remotethumbstick (Autodesk Fusion 360 design; units mm, degrees)
Autodesk Fusion 360 part; units mm, degrees
note: some values were not read from the file. Chosen so that the rebuilt part matches the saved one: which face or edge a step refers to.
sketch "Sketch1" plane through (0, 0, 0) normal (0, 1, 0) x (1, 0, 0)
  line L0 (0, 0) -> (-13.2, 0)
  line L1 (-13.2, 0) -> (-13.2, -13.2)
  line L2 (-13.2, -13.2) -> (0, -13.2)
  line L3 (0, -13.2) -> (0, 0)
  dimension "d1" = 13.2
  dimension "d2" = 13.2
  constraint horizontal L0
  constraint vertical L1
  constraint horizontal L2
  constraint vertical L3
  constraint coincident L0.start L3.end
  measures "d1" distance of L1.end L2.end
  measures "d2" distance of L0.end L1.end
extrude "Extrude1" add sketch "Sketch1" along normal blind 12 makes body 1
sketch "Sketch3" plane through (0, 0, 0) normal (0, 0, -1) x (1, 0, 0)
  line L0 (0, 0) -> (-13.2, 0)
  line L1 (-13.2, 0) -> (-13.2, -12)
  line L2 (-13.2, -12) -> (0, -12)
  line L3 (0, -12) -> (0, 0)
  line L4 (-11.4, 0) -> (-1.8, 0)
  line L5 (-1.8, 0) -> (-1.8, -12)
  line L6 (-1.8, -12) -> (-11.4, -12)
  line L7 (-11.4, -12) -> (-11.4, 0)
  dimension "d10" = 9.6
  dimension "d11" = 1.8
  constraint horizontal L4
  constraint vertical L5
  constraint horizontal L6
  constraint vertical L7
  constraint coincident L2 L5.end
  constraint coincident L0 L4.start
  measures "d10" distance of L4.start L4.end
  measures "d11" distance of L3 L5
extrude "Extrude3" add sketch "Sketch3" along normal blind 3 contours L0 L2 L4 L5 L6 L7 bodies 1
sketch "Sketch4" plane through (-13.2, 0, 0) normal (-1, 0, 0) x (0, -1, 0)
  line L0 (0, 0) -> (0, 13.2)
  line L1 (0, 13.2) -> (-12, 13.2)
  line L2 (-12, 13.2) -> (-12, 0)
  line L3 (-12, 0) -> (0, 0)
  line L4 (-12, 11.4) -> (0, 11.4)
  line L5 (0, 11.4) -> (0, 1.8)
  line L6 (0, 1.8) -> (-12, 1.8)
  line L7 (-12, 1.8) -> (-12, 11.4)
  dimension "d14" = 1.8
  dimension "d15" = 1.8
  constraint horizontal L4
  constraint vertical L5
  constraint horizontal L6
  constraint vertical L7
  constraint coincident L0 L5.end
  constraint coincident L2 L4.start
  measures "d14" distance of L1 L4
  measures "d15" distance of L3 L6
extrude "Extrude4" add sketch "Sketch4" along normal blind 3 contours L0 L2 L4 L5 L6 L7 bodies 1
sketch "Sketch6" plane through (0, 0, 13.2) normal (0, 0, 1) x (-1, 0, 0)
  line L0 (13.2, 0) -> (0, 0)
  line L1 (0, 0) -> (0, -12)
  line L2 (0, -12) -> (13.2, -12)
  line L3 (13.2, -12) -> (13.2, 0)
  line L4 (10.9, 0) -> (2.3, 0)
  line L5 (2.3, 0) -> (2.3, -5)
  line L6 (2.3, -5) -> (10.9, -5)
  line L7 (10.9, -5) -> (10.9, 0)
  dimension "d22" = 5
  dimension "d23" = 8.6
  dimension "d24" = 2.3
  constraint horizontal L4
  constraint vertical L5
  constraint horizontal L6
  constraint vertical L7
  constraint coincident L0 L4.start
  measures "d22" distance of L4.start L6.end
  measures "d23" distance of L4.start L4.end
  measures "d24" distance of L3 L7
extrude "Extrude6" [suppressed]
sketch "Sketch7" plane through (-10.9, 0, 0) normal (-1, 0, 0) x (0, -1, 0)
  line L0 (-5, 13.2) -> (0, 13.2)
  line L1 (0, 13.2) -> (0, 18.2)
  line L2 (0, 18.2) -> (-5, 18.2)
  line L3 (-5, 18.2) -> (-5, 13.2)
  line L4 (-5, 16.8629) -> (-8.201, 13.1133)
  line L5 (-5, 16.8629) -> (-5, 13.2)
  line L6 (-8.201, 13.1133) -> (-5, 13.2)
  point P0 (-12, 13.2)
  dimension "d27" = 3.8
  constraint coincident L3 L4.start
  constraint coincident L0.start L3.end
  measures "d27" distance of L4.end P0
extrude "Extrude7" [suppressed]
sketch "Sketch8" plane through (0, 0, 0) normal (1, 0, 0) x (0, 1, 0)
  line L0 (0, 13.2) -> (0, 0)
  line L1 (0, 0) -> (12, 0)
  line L2 (12, 0) -> (12, 13.2)
  line L3 (12, 13.2) -> (0, 13.2)
  line L4 (0, 10.9) -> (5, 10.9)
  line L5 (5, 10.9) -> (5, 2.3)
  line L6 (5, 2.3) -> (0, 2.3)
  line L7 (0, 2.3) -> (0, 10.9)
  dimension "d30" = 8.6
  dimension "d31" = 2.3
  dimension "d34" = 5
  constraint horizontal L4
  constraint vertical L5
  constraint horizontal L6
  constraint vertical L7
  constraint coincident L0 L4.start
  measures "d30" distance of L4.start L6.end
  measures "d31" distance of L3 L4
  measures "d34" distance of L5.end L6.end
extrude "Extrude8" add sketch "Sketch8" along normal blind 5 contours L0 L4 L5 L6 L7 bodies 1
sketch "Sketch9" plane through (0, 0, 10.9) normal (0, 0, 1) x (-1, 0, 0)
  line L0 (0, -5) -> (0, 0)
  line L1 (0, 0) -> (-5, 0)
  line L2 (-5, 0) -> (-5, -5)
  line L3 (-5, -5) -> (0, -5)
  line L4 (-3.7501, -5) -> (0, -8.4788)
  line L5 (0, -8.4788) -> (0, -5)
  line L6 (-3.7501, -5) -> (0, -5)
  constraint coincident L3 L4.start
  constraint coincident L0.start L3.end
  constraint perpendicular L3 L5
extrude "Extrude9" add sketch "Sketch9" against normal blind 8.6 contours L3 L4 L5 L6 bodies 1
sketch "Sketch10" plane through (0, 12, 0) normal (0, 1, 0) x (-1, 0, 0)
  line L0 (0, 13.2) -> (0, 0)
  line L1 (0, 0) -> (1.8, 0)
  line L2 (1.8, 0) -> (1.8, -3)
  line L3 (1.8, -3) -> (11.4, -3)
  line L4 (11.4, -3) -> (11.4, 0)
  line L5 (11.4, 0) -> (13.2, 0)
  line L6 (13.2, 0) -> (13.2, 1.8)
  line L7 (13.2, 1.8) -> (16.2, 1.8)
  line L8 (16.2, 1.8) -> (16.2, 11.4)
  line L9 (16.2, 11.4) -> (13.2, 11.4)
  line L10 (13.2, 11.4) -> (13.2, 13.2)
  line L11 (13.2, 13.2) -> (0, 13.2)
  line L12 (5.15, 8.55) -> (8.05, 8.55)
  line L13 (8.05, 8.55) -> (8.05, 4.65)
  line L14 (8.05, 4.65) -> (5.15, 4.65)
  line L15 (5.15, 4.65) -> (5.15, 8.55)
  line L16 (6.6, 8.55) -> (5.15, 4.65)
  line L17 (8.05, 4.65) -> (6.6, 8.55)
  line L18 (5.4515, 5.4609) -> (7.7485, 5.4609)
  dimension "d37" = 2.9
  dimension "d38" = 3.9
  dimension "d39" = 5.15
  dimension "d40" = 4.65
  constraint horizontal L12
  constraint vertical L13
  constraint horizontal L14
  constraint vertical L15
  constraint midpoint L12 L16.start
  constraint coincident L16 L18.start
  constraint coincident L17 L18.end
  constraint perpendicular L13 L18
  measures "d37" distance of L12.start L12.end
  measures "d38" distance of L12.start L14.end
  measures "d39" distance of L0 L15
  measures "d40" distance of L5 L14
extrude "Extrude10" add sketch "Sketch10" along normal blind 7.7 separate body contours L12 L15 L16 | L12 L13 L17 | L14 L16 L17 L18 makes body 2
